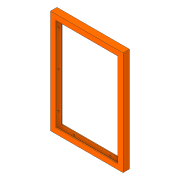
# Autodesk Inventor part: honeyCombFrame
Saved by Autodesk Inventor 2017 (Build 210142000, 142)
## iProperties
Created: 2016-12-01
Part Number: honeyCombFrame
Material: Generic
Document SubType Name: Modeling
Designer: krosie
Density: 1 g/cm^3
Appearance: Default
Author: krosie
Autodesk Inventor part; units mm, degrees
note: some values were not read from the file. Chosen so that the rebuilt part matches the saved one: direction of "Hole1"; direction of "Hole2".
ref_plane "YZ Plane" through (0, 0, 0) normal (1, 0, 0) x (0, 1, 0)
ref_plane "XZ Plane" through (0, 0, 0) normal (0, 1, 0) x (-1, 0, 0)
ref_plane "XY Plane" through (0, 0, 0) normal (0, 0, 1) x (1, 0, 0)
sketch "Sketch1" plane through (0, 0, 0) normal (0, 1, 0) x (-1, 0, 0)
  line L0 (-88.9, 127) -> (88.9, 127)
  line L1 (88.9, 127) -> (88.9, -127)
  line L2 (88.9, -127) -> (-88.9, -127)
  line L3 (-88.9, -127) -> (-88.9, 127)
  line L4 (-88.9, 127) -> (88.9, -127) construction
  line L5 (88.9, 127) -> (-88.9, -127) construction
  line L6 (75.9, 114) -> (-75.9, 114)
  line L7 (-75.9, 114) -> (-75.9, -114)
  line L8 (-75.9, -114) -> (75.9, -114)
  line L9 (75.9, -114) -> (75.9, 114)
  point P0 (0, 0)
  dimension "d1" = 254
  dimension "d2" = 177.8
  dimension "d3" = 13
  constraints: 20 end point, 4 parallel, 2 midpoint, 2 perpendicular, 1 horizontal, 3 other
  measures "d1" distance of L0.end L1.end
  measures "d2" distance of L1.end L2.end
  measures "d3" distance between parallel lines of L0 L6
extrude "Extrusion1" add sketch "Sketch1" along normal blind 15.875
shell "Shell1" thickness 2.3622 removed faces 4 at (-75.9, 5.2917, -38) at (25.3, 5.2917, -114) at (75.9, 5.2917, 38) at (-25.3, 5.2917, 114)
hole "Hole1" at (82.25, 15.875, 0) direction (0, -1, 0) diameter 4.496 end up to surface clearance for "Flat Head Machine Screw (82)" size "#8" standard "Ansi Unified Screw Threads"
pattern_linear "Rectangular Pattern1" count 3 spacing 88.9 along (0, 0, 1) of "Hole1" first direction both ways yes
mirror "Mirror1" about plane through (0, 0, 0) normal (1, 0, 0) of "Hole1", "Rectangular Pattern1"
hole "Hole2" at (44.45, 15.875, 120.65) direction (0, -1, 0) diameter 4.496 end up to surface clearance for "Flat Head Machine Screw (82)" size "#8" standard "Ansi Unified Screw Threads"
mirror "Mirror2" about plane through (0, 0, 0) normal (1, 0, 0) of "Hole2"
mirror "Mirror3" about plane through (0, 0, 0) normal (0, 0, 1) of "Hole2", "Mirror2"
body "Solid1"
